Autodesk Inventor part; units mm, degrees
(part 2 of 6)
  arc A552 (-21.7306, 49.25) -> (-21.2315, 49.5618) centre (-21.7304, 49.805) ccw
  arc A553 (-21.2315, 49.5618) -> (-21.1389, 49.8696) centre (-22.1304, 50) ccw
  arc A554 (-20.9902, 50) -> (-21.1389, 49.8696) centre (-20.9902, 49.85) ccw
  line L94 (-20.9902, 50) -> (-20.4709, 50)
  arc A555 (-20.3222, 49.8696) -> (-20.4709, 50) centre (-20.4709, 49.85) ccw
  arc A556 (-20.3222, 49.8696) -> (-20.2296, 49.5618) centre (-19.3307, 50) ccw
  arc A557 (-20.2296, 49.5618) -> (-19.7306, 49.25) centre (-19.7307, 49.805) ccw
  arc A558 (-19.7306, 49.25) -> (-19.2315, 49.5618) centre (-19.7304, 49.805) ccw
  arc A559 (-19.2315, 49.5618) -> (-19.1389, 49.8696) centre (-20.1304, 50) ccw
  arc A560 (-18.9902, 50) -> (-19.1389, 49.8696) centre (-18.9902, 49.85) ccw
  line L95 (-18.9902, 50) -> (-18.4709, 50)
  arc A561 (-18.3222, 49.8696) -> (-18.4709, 50) centre (-18.4709, 49.85) ccw
  arc A562 (-18.3222, 49.8696) -> (-18.2296, 49.5618) centre (-17.3307, 50) ccw
  arc A563 (-18.2296, 49.5618) -> (-17.7306, 49.25) centre (-17.7307, 49.805) ccw
  arc A564 (-17.7306, 49.25) -> (-17.2315, 49.5618) centre (-17.7304, 49.805) ccw
  arc A565 (-17.2315, 49.5618) -> (-17.1389, 49.8696) centre (-18.1304, 50) ccw
  arc A566 (-16.9902, 50) -> (-17.1389, 49.8696) centre (-16.9902, 49.85) ccw
  line L96 (-16.9902, 50) -> (-16.4709, 50)
  arc A567 (-16.3222, 49.8696) -> (-16.4709, 50) centre (-16.4709, 49.85) ccw
  arc A568 (-16.3222, 49.8696) -> (-16.2296, 49.5618) centre (-15.3307, 50) ccw
  arc A569 (-16.2296, 49.5618) -> (-15.7306, 49.25) centre (-15.7307, 49.805) ccw
  arc A570 (-15.7306, 49.25) -> (-15.2315, 49.5618) centre (-15.7304, 49.805) ccw
  arc A571 (-15.2315, 49.5618) -> (-15.1389, 49.8696) centre (-16.1304, 50) ccw
  arc A572 (-14.9902, 50) -> (-15.1389, 49.8696) centre (-14.9902, 49.85) ccw
  line L97 (-14.9902, 50) -> (-14.4709, 50)
  arc A573 (-14.3222, 49.8696) -> (-14.4709, 50) centre (-14.4709, 49.85) ccw
  arc A574 (-14.3222, 49.8696) -> (-14.2296, 49.5618) centre (-13.3307, 50) ccw
  arc A575 (-14.2296, 49.5618) -> (-13.7306, 49.25) centre (-13.7307, 49.805) ccw
  arc A576 (-13.7306, 49.25) -> (-13.2315, 49.5618) centre (-13.7304, 49.805) ccw
  arc A577 (-13.2315, 49.5618) -> (-13.1389, 49.8696) centre (-14.1304, 50) ccw
  arc A578 (-12.9902, 50) -> (-13.1389, 49.8696) centre (-12.9902, 49.85) ccw
  line L98 (-12.9902, 50) -> (-12.4709, 50)
  arc A579 (-12.3222, 49.8696) -> (-12.4709, 50) centre (-12.4709, 49.85) ccw
  arc A580 (-12.3222, 49.8696) -> (-12.2296, 49.5618) centre (-11.3307, 50) ccw
  arc A581 (-12.2296, 49.5618) -> (-11.7306, 49.25) centre (-11.7307, 49.805) ccw
  arc A582 (-11.7306, 49.25) -> (-11.2315, 49.5618) centre (-11.7304, 49.805) ccw
  arc A583 (-11.2315, 49.5618) -> (-11.1389, 49.8696) centre (-12.1304, 50) ccw
  arc A584 (-10.9902, 50) -> (-11.1389, 49.8696) centre (-10.9902, 49.85) ccw
  line L99 (-10.9902, 50) -> (-10.4709, 50)
  arc A585 (-10.3222, 49.8696) -> (-10.4709, 50) centre (-10.4709, 49.85) ccw
  arc A586 (-10.3222, 49.8696) -> (-10.2296, 49.5618) centre (-9.3307, 50) ccw
  arc A587 (-10.2296, 49.5618) -> (-9.7306, 49.25) centre (-9.7307, 49.805) ccw
  arc A588 (-9.7306, 49.25) -> (-9.2315, 49.5618) centre (-9.7304, 49.805) ccw
  arc A589 (-9.2315, 49.5618) -> (-9.1389, 49.8696) centre (-10.1304, 50) ccw
  arc A590 (-8.9902, 50) -> (-9.1389, 49.8696) centre (-8.9902, 49.85) ccw
  line L100 (-8.9902, 50) -> (-8.4709, 50)
  arc A591 (-8.3222, 49.8696) -> (-8.4709, 50) centre (-8.4709, 49.85) ccw
  arc A592 (-8.3222, 49.8696) -> (-8.2296, 49.5618) centre (-7.3307, 50) ccw
  arc A593 (-8.2296, 49.5618) -> (-7.7306, 49.25) centre (-7.7307, 49.805) ccw
  arc A594 (-7.7306, 49.25) -> (-7.2315, 49.5618) centre (-7.7304, 49.805) ccw
  arc A595 (-7.2315, 49.5618) -> (-7.1389, 49.8696) centre (-8.1304, 50) ccw
  arc A596 (-6.9902, 50) -> (-7.1389, 49.8696) centre (-6.9902, 49.85) ccw
  line L101 (-6.9902, 50) -> (-6.4709, 50)
  arc A597 (-6.3222, 49.8696) -> (-6.4709, 50) centre (-6.4709, 49.85) ccw
  arc A598 (-6.3222, 49.8696) -> (-6.2296, 49.5618) centre (-5.3307, 50) ccw
  arc A599 (-6.2296, 49.5618) -> (-5.7306, 49.25) centre (-5.7307, 49.805) ccw
  arc A600 (-5.7306, 49.25) -> (-5.2315, 49.5618) centre (-5.7304, 49.805) ccw
  arc A601 (-5.2315, 49.5618) -> (-5.1389, 49.8696) centre (-6.1304, 50) ccw
  arc A602 (-4.9902, 50) -> (-5.1389, 49.8696) centre (-4.9902, 49.85) ccw
  line L102 (-4.9902, 50) -> (-4.4709, 50)
  arc A603 (-4.3222, 49.8696) -> (-4.4709, 50) centre (-4.4709, 49.85) ccw
  arc A604 (-4.3222, 49.8696) -> (-4.2296, 49.5618) centre (-3.3307, 50) ccw
  arc A605 (-4.2296, 49.5618) -> (-3.7306, 49.25) centre (-3.7307, 49.805) ccw
  arc A606 (-3.7306, 49.25) -> (-3.2315, 49.5618) centre (-3.7304, 49.805) ccw
  arc A607 (-3.2315, 49.5618) -> (-3.1389, 49.8696) centre (-4.1304, 50) ccw
  arc A608 (-2.9902, 50) -> (-3.1389, 49.8696) centre (-2.9902, 49.85) ccw
  line L103 (-2.9902, 50) -> (-2.4709, 50)
  arc A609 (-2.3222, 49.8696) -> (-2.4709, 50) centre (-2.4709, 49.85) ccw
  arc A610 (-2.3222, 49.8696) -> (-2.2296, 49.5618) centre (-1.3307, 50) ccw
  arc A611 (-2.2296, 49.5618) -> (-1.7306, 49.25) centre (-1.7307, 49.805) ccw
  arc A612 (-1.7306, 49.25) -> (-1.2315, 49.5618) centre (-1.7304, 49.805) ccw
  arc A613 (-1.2315, 49.5618) -> (-1.1389, 49.8696) centre (-2.1304, 50) ccw
  arc A614 (-0.9902, 50) -> (-1.1389, 49.8696) centre (-0.9902, 49.85) ccw
  line L104 (-0.9902, 50) -> (-0.3754, 50)
  arc A615 (-0.3433, 49.9187) -> (-0.3754, 50) centre (-0.4928, 49.9067) ccw
  arc A616 (-0.3433, 49.9187) -> (-0.2664, 49.6066) centre (0.6535, 49.9986) ccw
  arc A617 (-0.2664, 49.6066) -> (0.2388, 49.2692) centre (0.2441, 49.8242) ccw
  arc A618 (0.2388, 49.2692) -> (0.7304, 49.556) centre (0.2445, 49.8242) ccw
  arc A619 (0.7304, 49.556) -> (0.8385, 49.8586) centre (-0.1451, 50.0392) ccw
  arc A620 (0.9717, 49.9809) -> (0.8385, 49.8586) centre (0.986, 49.8316) ccw
  arc A621 (1.534, 49.9523) -> (0.9717, 49.9809) centre (0, 25.315) ccw
  arc A622 (1.6541, 49.8172) -> (1.534, 49.9523) centre (1.5046, 49.8052) ccw
  arc A623 (1.6541, 49.8172) -> (1.731, 49.5051) centre (2.6509, 49.8971) ccw
  arc A624 (1.731, 49.5051) -> (2.191, 49.17) centre (2.2415, 49.7227) ccw
  arc A625 (2.191, 49.17) -> (2.7278, 49.4544) centre (2.2419, 49.7227) ccw
  arc A626 (2.7278, 49.4544) -> (2.8359, 49.7571) centre (1.8523, 49.9377) ccw
  arc A627 (2.8736, 49.8322) -> (2.8359, 49.7571) centre (2.9834, 49.73) ccw
  arc A628 (3.5639, 49.7414) -> (2.8736, 49.8322) centre (0, 25.315) ccw
  arc A629 (3.5809, 49.6591) -> (3.5639, 49.7414) centre (3.4314, 49.6711) ccw
  arc A630 (3.5809, 49.6591) -> (3.6071, 49.3388) centre (4.5777, 49.5792) ccw
  arc A631 (3.6071, 49.3388) -> (4.0521, 48.9252) centre (4.1458, 49.4722) ccw
  arc A632 (4.0521, 48.9252) -> (4.5831, 49.13) centre (4.1461, 49.4722) ccw
  arc A633 (4.5831, 49.13) -> (4.738, 49.4116) centre (3.7958, 49.7466) ccw
  arc A634 (4.889, 49.511) -> (4.738, 49.4116) centre (4.8793, 49.3613) ccw
  arc A635 (5.4396, 49.3932) -> (4.889, 49.511) centre (0, 25.315) ccw
  arc A636 (5.5366, 49.2407) -> (5.4396, 49.3932) centre (5.3871, 49.2527) ccw
  arc A637 (5.5366, 49.2407) -> (5.5628, 48.9204) centre (6.5335, 49.1608) ccw
  arc A638 (5.5628, 48.9204) -> (5.9635, 48.5162) centre (6.1015, 49.0538) ccw
  arc A639 (5.9635, 48.5162) -> (6.5388, 48.7115) centre (6.1019, 49.0537) ccw
  arc A640 (6.5388, 48.7115) -> (6.6937, 48.9931) centre (5.7515, 49.3281) ccw
  arc A641 (6.7429, 49.0612) -> (6.6937, 48.9931) centre (6.8351, 48.9429) ccw
  arc A642 (7.41, 48.8616) -> (6.7429, 49.0612) centre (0, 25.315) ccw
  arc A643 (7.4136, 48.7777) -> (7.41, 48.8616) centre (7.2679, 48.8133) ccw
  arc A644 (7.4136, 48.7777) -> (7.3884, 48.4573) centre (8.385, 48.54) ccw
  arc A645 (7.3884, 48.4573) -> (7.7618, 47.9781) centre (7.9415, 48.5032) ccw
  arc A646 (7.7618, 47.9781) -> (8.3187, 48.0956) centre (7.9418, 48.5031) ccw
  arc A647 (8.3187, 48.0956) -> (8.5165, 48.3489) centre (7.6397, 48.8298) ccw
  arc A648 (8.6814, 48.4231) -> (8.5165, 48.3489) centre (8.648, 48.2768) ccw
  arc A649 (9.2062, 48.219) -> (8.6814, 48.4231) centre (0, 25.315) ccw
  arc A650 (9.2777, 48.053) -> (9.2062, 48.219) centre (9.132, 48.0887) ccw
  arc A651 (9.2777, 48.053) -> (9.2525, 47.7326) centre (10.2491, 47.8153) ccw
  arc A652 (9.2525, 47.7326) -> (9.5837, 47.2698) centre (9.8056, 47.7785) ccw
  arc A653 (9.5837, 47.2698) -> (10.1828, 47.3709) centre (9.8059, 47.7784) ccw
  arc A654 (10.1828, 47.3709) -> (10.3806, 47.6243) centre (9.5038, 48.1051) ccw
  arc A655 (10.44, 47.6836) -> (10.3806, 47.6243) centre (10.5121, 47.5521) ccw
  arc A656 (11.0667, 47.3803) -> (10.44, 47.6836) centre (0, 25.315) ccw
  arc A657 (11.057, 47.2969) -> (11.0667, 47.3803) centre (10.9188, 47.3553) ccw
  arc A658 (11.057, 47.2969) -> (10.981, 46.9846) centre (11.978, 46.9075) ccw
  arc A659 (10.981, 46.9846) -> (11.2734, 46.452) centre (11.5344, 46.9418) ccw
  arc A660 (11.2734, 46.452) -> (11.8418, 46.4794) centre (11.5347, 46.9416) ccw
  arc A661 (11.8418, 46.4794) -> (12.0775, 46.6979) centre (11.2884, 47.3123) ccw
  arc A662 (12.252, 46.7448) -> (12.0775, 46.6979) centre (12.1958, 46.6058) ccw
  arc A663 (12.7377, 46.4598) -> (12.252, 46.7448) centre (0, 25.315) ccw
  arc A664 (12.7818, 46.2845) -> (12.7377, 46.4598) centre (12.6436, 46.3429) ccw
  arc A665 (12.7818, 46.2845) -> (12.7059, 45.9722) centre (13.7029, 45.8951) ccw
  arc A666 (12.7059, 45.9722) -> (12.9591, 45.4625) centre (13.2592, 45.9294) ccw
  arc A667 (12.9591, 45.4625) -> (13.5666, 45.4669) centre (13.2595, 45.9292) ccw
  arc A668 (13.5666, 45.4669) -> (13.8023, 45.6855) centre (13.0133, 46.2999) ccw
  arc A669 (13.8704, 45.7347) -> (13.8023, 45.6855) centre (13.9206, 45.5933) ccw
  arc A670 (14.4408, 45.3353) -> (13.8704, 45.7347) centre (0, 25.315) ccw
  arc A671 (14.4179, 45.2545) -> (14.4408, 45.3353) centre (14.2908, 45.3342) ccw
  arc A672 (14.4179, 45.2545) -> (14.2931, 44.9583) centre (15.2651, 44.7234) ccw
  arc A673 (14.2931, 44.9583) -> (14.4969, 44.386) centre (14.8326, 44.8279) ccw
  arc A674 (14.4969, 44.386) -> (15.0624, 44.3224) centre (14.8329, 44.8277) ccw
  arc A675 (15.0624, 44.3224) -> (15.3299, 44.5006) centre (14.6488, 45.2329) ccw
  arc A676 (15.5097, 44.5191) -> (15.3299, 44.5006) centre (15.432, 44.3908) ccw
  arc A677 (15.9437, 44.1604) -> (15.5097, 44.5191) centre (0, 25.315) ccw
  arc A678 (15.9594, 43.9803) -> (15.9437, 44.1604) centre (15.8323, 44.0599) ccw
  arc A679 (15.9594, 43.9803) -> (15.8346, 43.6841) centre (16.8066, 43.4491) ccw
  arc A680 (15.8346, 43.6841) -> (16.0035, 43.1406) centre (16.3741, 43.5537) ccw
  arc A681 (16.0035, 43.1406) -> (16.6039, 43.0481) centre (16.3744, 43.5534) ccw
  arc A682 (16.6039, 43.0481) -> (16.8714, 43.2263) centre (16.1903, 43.9586) ccw
  arc A683 (16.9464, 43.264) -> (16.8714, 43.2263) centre (16.9735, 43.1165) ccw
  arc A684 (17.4459, 42.7789) -> (16.9464, 43.264) centre (0, 25.315) ccw
  arc A685 (17.4104, 42.7028) -> (17.4459, 42.7789) centre (17.2977, 42.8017) ccw
  arc A686 (17.4104, 42.7028) -> (17.2401, 42.4303) centre (18.1623, 42.0435) ccw
  arc A687 (17.2401, 42.4303) -> (17.3501, 41.8328) centre (17.7519, 42.2156) ccw
  arc A688 (17.3501, 41.8328) -> (17.8983, 41.6799) centre (17.7522, 42.2153) ccw
  arc A689 (17.8983, 41.6799) -> (18.1907, 41.8132) centre (17.635, 42.6446) ccw
  arc A690 (18.3712, 41.8029) -> (18.1907, 41.8132) centre (18.274, 41.6885) ccw
  arc A691 (18.7425, 41.3795) -> (18.3712, 41.8029) centre (0, 25.315) ccw
  arc A692 (18.7292, 41.1992) -> (18.7425, 41.3795) centre (18.6165, 41.2981) ccw
  arc A693 (18.7292, 41.1992) -> (18.5589, 40.9267) centre (19.4811, 40.5399) ccw
  arc A694 (18.5589, 40.9267) -> (18.639, 40.3632) centre (19.0707, 40.712) ccw
  arc A695 (18.639, 40.3632) -> (19.2171, 40.1763) centre (19.0709, 40.7117) ccw
  arc A696 (19.2171, 40.1763) -> (19.5095, 40.3097) centre (18.9538, 41.141) ccw
  arc A697 (19.5896, 40.3349) -> (19.5095, 40.3097) centre (19.5928, 40.1849) ccw
  arc A698 (20.0054, 39.7764) -> (19.5896, 40.3349) centre (0, 25.315) ccw
  arc A699 (19.9583, 39.7069) -> (20.0054, 39.7764) centre (19.8627, 39.8225) ccw
  arc A700 (19.9583, 39.7069) -> (19.7467, 39.465) centre (20.5954, 38.9362) ccw
  arc A701 (19.7467, 39.465) -> (19.76, 38.8576) centre (20.2177, 39.1715) ccw
  arc A702 (19.76, 38.8576) -> (20.2769, 38.6194) centre (20.2179, 39.1712) ccw
  arc A703 (20.2769, 38.6194) -> (20.5868, 38.7044) centre (20.1707, 39.6137) ccw
  arc A704 (20.7633, 38.6654) -> (20.5868, 38.7044) centre (20.6492, 38.568) ccw
  arc A705 (21.0624, 38.1883) -> (20.7633, 38.6654) centre (0, 25.315) ccw
  arc A706 (21.0207, 38.0124) -> (21.0624, 38.1883) centre (20.9251, 38.1281) ccw
  arc A707 (21.0207, 38.0124) -> (20.8091, 37.7705) centre (21.6578, 37.2417) ccw
  arc A708 (20.8091, 37.7705) -> (20.7984, 37.2015) centre (21.2802, 37.477) ccw
  arc A709 (20.7984, 37.2015) -> (21.3393, 36.9249) centre (21.2803, 37.4767) ccw
  arc A710 (21.3393, 36.9249) -> (21.6492, 37.0099) centre (21.2331, 37.9192) ccw
  arc A711 (21.7323, 37.0221) -> (21.6492, 37.0099) centre (21.7116, 36.8735) ccw
  arc A712 (22.0539, 36.4045) -> (21.7323, 37.0221) centre (0, 25.315) ccw
  arc A713 (21.9962, 36.3434) -> (22.0539, 36.4045) centre (21.9203, 36.4728) ccw
  arc A714 (21.9962, 36.3434) -> (21.7488, 36.1383) centre (22.5025, 35.481) ccw
  arc A715 (21.7488, 36.1383) -> (21.6652, 35.5365) centre (22.1671, 35.7735) ccw
  arc A716 (21.6652, 35.5365) -> (22.1375, 35.219) centre (22.1673, 35.7732) ccw
  arc A717 (22.1375, 35.219) -> (22.457, 35.2535) centre (22.1911, 36.2175) ccw
  arc A718 (22.6251, 35.1869) -> (22.457, 35.2535) centre (22.4969, 35.1089) ccw
  arc A719 (22.8444, 34.6683) -> (22.6251, 35.1869) centre (0, 25.315) ccw
  arc A720 (22.7751, 34.5013) -> (22.8444, 34.6683) centre (22.6992, 34.6306) ccw
  arc A721 (22.7751, 34.5013) -> (22.5277, 34.2962) centre (23.2814, 33.6389) ccw
  arc A722 (22.5277, 34.2962) -> (22.4265, 33.7361) centre (22.946, 33.9314) ccw
  arc A723 (22.4265, 33.7361) -> (22.9164, 33.3768) centre (22.9461, 33.931) ccw
  arc A724 (22.9164, 33.3768) -> (23.2359, 33.4114) centre (22.9699, 34.3754) ccw
  arc A725 (23.3199, 33.4102) -> (23.2359, 33.4114) centre (23.2758, 33.2668) ccw
  arc A726 (23.5389, 32.7493) -> (23.3199, 33.4102) centre (0, 25.315) ccw
  arc A727 (23.4723, 32.6981) -> (23.5389, 32.7493) centre (23.4179, 32.8379) ccw
  arc A728 (23.4723, 32.6981) -> (23.1954, 32.535) centre (23.8347, 31.7661) ccw
  arc A729 (23.1954, 32.535) -> (23.017, 31.9543) centre (23.5502, 32.1083) ccw
  arc A730 (23.017, 31.9543) -> (23.4326, 31.5655) centre (23.5503, 32.1079) ccw
  arc A731 (23.4326, 31.5655) -> (23.7536, 31.5488) centre (23.6446, 32.5428) ccw
  arc A732 (23.9089, 31.4562) -> (23.7536, 31.5488) centre (23.7699, 31.3997) ccw
  arc A733 (24.0427, 30.9093) -> (23.9089, 31.4562) centre (0, 25.315) ccw
  arc A734 (23.9478, 30.7555) -> (24.0427, 30.9093) centre (23.8934, 30.8953) ccw
  arc A735 (23.9478, 30.7555) -> (23.6708, 30.5924) centre (24.3101, 29.8234) ccw
  arc A736 (23.6708, 30.5924) -> (23.4817, 30.0556) centre (24.0256, 30.1656) ccw
  arc A737 (23.4817, 30.0556) -> (23.9081, 29.6229) centre (24.0257, 30.1653) ccw
  arc A738 (23.9081, 29.6229) -> (24.229, 29.6061) centre (24.12, 30.6002) ccw
  arc A739 (24.3117, 29.5915) -> (24.229, 29.6061) centre (24.2454, 29.457) ccw
  arc A740 (24.4227, 28.9041) -> (24.3117, 29.5915) centre (0, 25.315) ccw
  arc A741 (24.3488, 28.8643) -> (24.4227, 28.9041) centre (24.3174, 29.0109) ccw
  arc A742 (24.3488, 28.8643) -> (24.0494, 28.7474) centre (24.558, 27.8864) ccw
  arc A743 (24.0494, 28.7474) -> (23.7808, 28.2025) centre (24.3317, 28.2695) ccw
  arc A744 (23.7808, 28.2025) -> (24.1292, 27.7525) centre (24.3317, 28.2692) ccw
  arc A745 (24.1292, 27.7525) -> (24.4434, 27.6848) centre (24.4941, 28.6835) ccw
  arc A746 (24.5819, 27.5687) -> (24.4434, 27.6848) centre (24.4357, 27.535) ccw
  arc A747 (24.6269, 27.0074) -> (24.5819, 27.5687) centre (0, 25.315) ccw
  arc A748 (24.5086, 26.8707) -> (24.6269, 27.0074) centre (24.4772, 27.0173) ccw
  arc A749 (24.5086, 26.8707) -> (24.2093, 26.7538) centre (24.7179, 25.8928) ccw
  arc A750 (24.2093, 26.7538) -> (23.937, 26.254) centre (24.4916, 26.2759) ccw
  arc A751 (23.937, 26.254) -> (24.289, 25.7589) centre (24.4916, 26.2756) ccw
  arc A752 (24.289, 25.7589) -> (24.6032, 25.6912) centre (24.654, 26.6899) ccw
  arc A753 (24.6825, 25.6636) -> (24.6032, 25.6912) centre (24.5956, 25.5414) ccw
  arc A754 (24.6826, 24.9673) -> (24.6825, 25.6636) centre (0, 25.315) ccw
  arc A755 (24.6032, 24.9397) -> (24.6826, 24.9673) centre (24.5956, 25.0895) ccw
  arc A756 (24.6032, 24.9397) -> (24.289, 24.872) centre (24.654, 23.941) ccw
  arc A757 (24.289, 24.872) -> (23.937, 24.3769) centre (24.4916, 24.3553) ccw
  arc A758 (23.937, 24.3769) -> (24.2093, 23.8771) centre (24.4916, 24.355) ccw
  arc A759 (24.2093, 23.8771) -> (24.5087, 23.7602) centre (24.7179, 24.7381) ccw
  arc A760 (24.627, 23.6235) -> (24.5087, 23.7602) centre (24.4773, 23.6136) ccw
  arc A761 (24.582, 23.0622) -> (24.627, 23.6235) centre (0, 25.315) ccw
  arc A762 (24.4434, 22.9461) -> (24.582, 23.0622) centre (24.4358, 23.0959) ccw
  arc A763 (24.4434, 22.9461) -> (24.1293, 22.8784) centre (24.4943, 21.9474) ccw
  arc A764 (24.1293, 22.8784) -> (23.7809, 22.4284) centre (24.3318, 22.3617) ccw
  arc A765 (23.7809, 22.4284) -> (24.0495, 21.8835) centre (24.3318, 22.3614) ccw
  arc A766 (24.0495, 21.8835) -> (24.3489, 21.7666) centre (24.5581, 22.7445) ccw
  arc A767 (24.4228, 21.7268) -> (24.3489, 21.7666) centre (24.3175, 21.62) ccw
  arc A768 (24.3119, 21.0394) -> (24.4228, 21.7268) centre (0, 25.315) ccw
  arc A769 (24.2292, 21.0248) -> (24.3119, 21.0394) centre (24.2455, 21.1739) ccw
  arc A770 (24.2292, 21.0248) -> (23.9082, 21.008) centre (24.1202, 20.0307) ccw
  arc A771 (23.9082, 21.008) -> (23.4818, 20.5753) centre (24.0259, 20.4656) ccw
  arc A772 (23.4818, 20.5753) -> (23.671, 20.0385) centre (24.0258, 20.4653) ccw
  arc A773 (23.671, 20.0385) -> (23.948, 19.8754) centre (24.3103, 20.8075) ccw
  arc A774 (24.0429, 19.7216) -> (23.948, 19.8754) centre (23.8936, 19.7356) ccw
  arc A775 (23.9091, 19.1747) -> (24.0429, 19.7216) centre (0, 25.315) ccw
  arc A776 (23.7538, 19.0821) -> (23.9091, 19.1747) centre (23.7702, 19.2312) ccw
  arc A777 (23.7538, 19.0821) -> (23.4329, 19.0653) centre (23.6449, 18.088) ccw
  arc A778 (23.4329, 19.0653) -> (23.0172, 18.6766) centre (23.5505, 18.5229) ccw
  arc A779 (23.0172, 18.6766) -> (23.1956, 18.0958) centre (23.5504, 18.5226) ccw
  arc A780 (23.1956, 18.0958) -> (23.4726, 17.9327) centre (23.8349, 18.8648) ccw
  arc A781 (23.5392, 17.8816) -> (23.4726, 17.9327) centre (23.4182, 17.7929) ccw
  arc A782 (23.3202, 17.2207) -> (23.5392, 17.8816) centre (0, 25.315) ccw
  arc A783 (23.2362, 17.2194) -> (23.3202, 17.2207) centre (23.2761, 17.364) ccw
  arc A784 (23.2362, 17.2194) -> (22.9167, 17.254) centre (22.9703, 16.2554) ccw
  arc A785 (22.9167, 17.254) -> (22.4268, 16.8947) centre (22.9464, 16.6998) ccw
  arc A786 (22.4268, 16.8947) -> (22.528, 16.3347) centre (22.9463, 16.6995) ccw
  arc A787 (22.528, 16.3347) -> (22.7754, 16.1295) centre (23.2817, 16.992) ccw
  arc A788 (22.8447, 15.9626) -> (22.7754, 16.1295) centre (22.6995, 16.0002) ccw
  arc A789 (22.6255, 15.4439) -> (22.8447, 15.9626) centre (0, 25.315) ccw
  arc A790 (22.4574, 15.3773) -> (22.6255, 15.4439) centre (22.4973, 15.5219) ccw
  arc A791 (22.4574, 15.3773) -> (22.1379, 15.4119) centre (22.1915, 14.4133) ccw
  arc A792 (22.1379, 15.4119) -> (21.6656, 15.0943) centre (22.1676, 14.8577) ccw
  arc A793 (21.6656, 15.0943) -> (21.7492, 14.4925) centre (22.1675, 14.8573) ccw
  arc A794 (21.7492, 14.4925) -> (21.9966, 14.2874) centre (22.5029, 15.1498) ccw
  arc A795 (22.0543, 14.2263) -> (21.9966, 14.2874) centre (21.9207, 14.1581) ccw
  arc A796 (21.7327, 13.6087) -> (22.0543, 14.2263) centre (0, 25.315) ccw
  arc A797 (21.6496, 13.6209) -> (21.7327, 13.6087) centre (21.7121, 13.7573) ccw
  arc A798 (21.6496, 13.6209) -> (21.3397, 13.7059) centre (21.2335, 12.7116) ccw
  arc A799 (21.3397, 13.7059) -> (20.7988, 13.4293) centre (21.2808, 13.1541) ccw
  arc A800 (20.7988, 13.4293) -> (20.8096, 12.8602) centre (21.2806, 13.1537) ccw
  arc A801 (20.8096, 12.8602) -> (21.0211, 12.6183) centre (21.6583, 13.3891) ccw
  arc A802 (21.0629, 12.4424) -> (21.0211, 12.6183) centre (20.9256, 12.5027) ccw
  arc A803 (20.7638, 11.9654) -> (21.0629, 12.4424) centre (0, 25.315) ccw
  arc A804 (20.5873, 11.9263) -> (20.7638, 11.9654) centre (20.6497, 12.0627) ccw
  arc A805 (20.5873, 11.9263) -> (20.2774, 12.0114) centre (20.1712, 11.017) ccw
  arc A806 (20.2774, 12.0114) -> (19.7605, 11.7731) centre (20.2184, 11.4595) ccw
  arc A807 (19.7605, 11.7731) -> (19.7472, 11.1657) centre (20.2182, 11.4592) ccw
  arc A808 (19.7472, 11.1657) -> (19.9588, 10.9238) centre (20.5959, 11.6945) ccw
  arc A809 (20.0059, 10.8543) -> (19.9588, 10.9238) centre (19.8632, 10.8082) ccw
  arc A810 (19.5901, 10.2958) -> (20.0059, 10.8543) centre (0, 25.315) ccw
  arc A811 (19.51, 10.3211) -> (19.5901, 10.2958) centre (19.5934, 10.4458) ccw
  arc A812 (19.51, 10.3211) -> (19.2176, 10.4544) centre (18.9544, 9.4897) ccw
  arc A813 (19.2176, 10.4544) -> (18.6395, 10.2674) centre (19.0715, 9.919) ccw
  arc A814 (18.6395, 10.2674) -> (18.5595, 9.704) centre (19.0713, 9.9187) ccw
  arc A815 (18.5595, 9.704) -> (18.7298, 9.4314) centre (19.4816, 10.0908) ccw
  arc A816 (18.7431, 9.2512) -> (18.7298, 9.4314) centre (18.6171, 9.3325) ccw
  arc A817 (18.3718, 8.8278) -> (18.7431, 9.2512) centre (0, 25.315) ccw
  arc A818 (18.1913, 8.8174) -> (18.3718, 8.8278) centre (18.2747, 8.9421) ccw
  arc A819 (18.1913, 8.8174) -> (17.8989, 8.9507) centre (17.6356, 7.986) ccw
  arc A820 (17.8989, 8.9507) -> (17.3507, 8.7979) centre (17.7528, 8.4153) ccw
  arc A821 (17.3507, 8.7979) -> (17.2407, 8.2004) centre (17.7525, 8.4151) ccw
  arc A822 (17.2407, 8.2004) -> (17.4111, 7.9278) centre (18.1629, 8.5872) ccw
  arc A823 (17.4466, 7.8517) -> (17.4111, 7.9278) centre (17.2983, 7.8289) ccw
  arc A824 (16.9471, 7.3666) -> (17.4466, 7.8517) centre (0, 25.315) ccw
  arc A825 (16.872, 7.4043) -> (16.9471, 7.3666) centre (16.9742, 7.5141) ccw
  arc A826 (16.872, 7.4043) -> (16.6046, 7.5825) centre (16.191, 6.672) ccw
  arc A827 (16.6046, 7.5825) -> (16.0041, 7.49) centre (16.375, 7.0772) ccw
  arc A828 (16.0041, 7.49) -> (15.8353, 6.9465) centre (16.3748, 7.0769) ccw
  arc A829 (15.8353, 6.9465) -> (15.9601, 6.6503) centre (16.8073, 7.1815) ccw
  arc A830 (15.9444, 6.4702) -> (15.9601, 6.6503) centre (15.833, 6.5706) ccw
  arc A831 (15.5104, 6.1114) -> (15.9444, 6.4702) centre (0, 25.315) ccw
  arc A832 (15.3306, 6.1299) -> (15.5104, 6.1114) centre (15.4327, 6.2398) ccw
  arc A833 (15.3306, 6.1299) -> (15.0631, 6.3081) centre (14.6496, 5.3977) ccw
  arc A834 (15.0631, 6.3081) -> (14.4976, 6.2446) centre (14.8336, 5.8028) ccw
  arc A835 (14.4976, 6.2446) -> (14.2938, 5.6722) centre (14.8333, 5.8026) ccw
  arc A836 (14.2938, 5.6722) -> (14.4186, 5.376) centre (15.2658, 5.9072) ccw
  arc A837 (14.4415, 5.2952) -> (14.4186, 5.376) centre (14.2915, 5.2963) ccw
  arc A838 (13.8711, 4.8959) -> (14.4415, 5.2952) centre (0, 25.315) ccw
  arc A839 (13.803, 4.945) -> (13.8711, 4.8959) centre (13.9214, 5.0372) ccw
  arc A840 (13.803, 4.945) -> (13.5674, 5.1636) centre (13.014, 4.3306) ccw
  arc A841 (13.5674, 5.1636) -> (12.9599, 5.168) centre (13.2603, 4.7013) ccw
  arc A842 (12.9599, 5.168) -> (12.7066, 4.6583) centre (13.26, 4.7011) ccw
  arc A843 (12.7066, 4.6583) -> (12.7826, 4.346) centre (13.7036, 4.7354) ccw
  arc A844 (12.7384, 4.1707) -> (12.7826, 4.346) centre (12.6444, 4.2876) ccw
  arc A845 (12.2528, 3.8856) -> (12.7384, 4.1707) centre (0, 25.315) ccw
  arc A846 (12.0782, 3.9325) -> (12.2528, 3.8856) centre (12.1966, 4.0247) ccw
  arc A847 (12.0782, 3.9325) -> (11.8426, 4.1511) centre (11.2892, 3.3181) ccw
  arc A848 (11.8426, 4.1511) -> (11.2741, 4.1784) centre (11.5355, 3.6888) ccw
  arc A849 (11.2741, 4.1784) -> (10.9818, 3.6458) centre (11.5352, 3.6886) ccw
  arc A850 (10.9818, 3.6458) -> (11.0578, 3.3335) centre (11.9788, 3.723) ccw
  arc A851 (11.0675, 3.2501) -> (11.0578, 3.3335) centre (10.9196, 3.2751) ccw
  arc A852 (10.4408, 2.9467) -> (11.0675, 3.2501) centre (0, 25.315) ccw
  arc A853 (10.3814, 3.0061) -> (10.4408, 2.9467) centre (10.5129, 3.0783) ccw
  arc A854 (10.3814, 3.0061) -> (10.1836, 3.2594) centre (9.5046, 2.5253) ccw
  arc A855 (10.1836, 3.2594) -> (9.5845, 3.3605) centre (9.8068, 2.852) ccw
  arc A856 (9.5845, 3.3605) -> (9.2533, 2.8977) centre (9.8064, 2.8518) ccw
  arc A857 (9.2533, 2.8977) -> (9.2786, 2.5773) centre (10.2499, 2.815) ccw
  arc A858 (9.2071, 2.4113) -> (9.2786, 2.5773) centre (9.1329, 2.5417) ccw
  arc A859 (8.6822, 2.2073) -> (9.2071, 2.4113) centre (0, 25.315) ccw
  arc A860 (8.5174, 2.2814) -> (8.6822, 2.2073) centre (8.6489, 2.3535) ccw
  arc A861 (8.5174, 2.2814) -> (8.3195, 2.5347) centre (7.6406, 1.8005) ccw
  arc A862 (8.3195, 2.5347) -> (7.7627, 2.6522) centre (7.9427, 2.1272) ccw
  arc A863 (7.7627, 2.6522) -> (7.3893, 2.173) centre (7.9424, 2.1271) ccw
  arc A864 (7.3893, 2.173) -> (7.4145, 1.8526) centre (8.3858, 2.0903) ccw
  arc A865 (7.4108, 1.7687) -> (7.4145, 1.8526) centre (7.2688, 1.8169) ccw
  arc A866 (6.7438, 1.569) -> (7.4108, 1.7687) centre (0, 25.315) ccw
  arc A867 (6.6946, 1.6371) -> (6.7438, 1.569) centre (6.8359, 1.6874) ccw
  arc A868 (6.6946, 1.6371) -> (6.5397, 1.9187) centre (5.7524, 1.3021) ccw
  arc A869 (6.5397, 1.9187) -> (5.9644, 2.114) centre (6.1027, 1.5765) ccw
  arc A870 (5.9644, 2.114) -> (5.5637, 1.7098) centre (6.1024, 1.5764) ccw
  arc A871 (5.5637, 1.7098) -> (5.5375, 1.3895) centre (6.5343, 1.4694) ccw
  arc A872 (5.4405, 1.237) -> (5.5375, 1.3895) centre (5.388, 1.3775) ccw
  arc A873 (4.8899, 1.1192) -> (5.4405, 1.237) centre (0, 25.315) ccw
  arc A874 (4.7389, 1.2186) -> (4.8899, 1.1192) centre (4.8802, 1.2689) ccw
  arc A875 (4.7389, 1.2186) -> (4.5839, 1.5002) centre (3.7967, 0.8836) ccw
  arc A876 (4.5839, 1.5002) -> (4.0529, 1.7049) centre (4.147, 1.158) ccw
  arc A877 (4.0529, 1.7049) -> (3.6079, 1.2913) centre (4.1467, 1.1579) ccw
  arc A878 (3.6079, 1.2913) -> (3.5818, 0.971) centre (4.5786, 1.0509) ccw
  arc A879 (3.5648, 0.8888) -> (3.5818, 0.971) centre (3.4323, 0.959) ccw
  arc A880 (2.8745, 0.7979) -> (3.5648, 0.8888) centre (0, 25.315) ccw
  arc A881 (2.8368, 0.873) -> (2.8745, 0.7979) centre (2.9843, 0.9001) ccw
  arc A882 (2.8368, 0.873) -> (2.7287, 1.1757) centre (1.8532, 0.6924) ccw
  arc A883 (2.7287, 1.1757) -> (2.1918, 1.4601) centre (2.2428, 0.9074) ccw
  arc A884 (2.1918, 1.4601) -> (1.7319, 1.1249) centre (2.2424, 0.9074) ccw
  arc A885 (1.7319, 1.1249) -> (1.655, 0.8129) centre (2.6518, 0.733) ccw
  arc A886 (1.5349, 0.6778) -> (1.655, 0.8129) centre (1.5055, 0.8249) ccw
  arc A887 (0.9726, 0.6492) -> (1.5349, 0.6778) centre (0, 25.315) ccw
  arc A888 (0.8394, 0.7714) -> (0.9726, 0.6492) centre (0.9869, 0.7985) ccw
  arc A889 (0.8394, 0.7714) -> (0.7313, 1.0741) centre (-0.1442, 0.5908) ccw
  arc A890 (0.7313, 1.0741) -> (0.2397, 1.3608) centre (0.2454, 0.8058) ccw
  arc A891 (0.2397, 1.3608) -> (-0.2656, 1.0234) centre (0.245, 0.8058) ccw
  arc A892 (-0.2656, 1.0234) -> (-0.3424, 0.7113) centre (0.6544, 0.6314) ccw
  arc A893 (-0.3744, 0.63) -> (-0.3424, 0.7113) centre (-0.4919, 0.7233) ccw
  line L105 (-0.3744, 0.63) -> (-0.9893, 0.63)
  arc A894 (-1.138, 0.7604) -> (-0.9893, 0.63) centre (-0.9893, 0.78) ccw
  arc A895 (-1.138, 0.7604) -> (-1.2306, 1.0682) centre (-2.1294, 0.63) ccw
  arc A896 (-1.2306, 1.0682) -> (-1.7296, 1.38) centre (-1.7294, 0.825) ccw
  arc A897 (-1.7296, 1.38) -> (-2.2287, 1.0682) centre (-1.7298, 0.825) ccw
  arc A898 (-2.2287, 1.0682) -> (-2.3213, 0.7604) centre (-1.3298, 0.63) ccw
  arc A899 (-2.47, 0.63) -> (-2.3213, 0.7604) centre (-2.47, 0.78) ccw
  line L106 (-2.47, 0.63) -> (-2.9893, 0.63)
  arc A900 (-3.138, 0.7604) -> (-2.9893, 0.63) centre (-2.9893, 0.78) ccw
  arc A901 (-3.138, 0.7604) -> (-3.2306, 1.0682) centre (-4.1294, 0.63) ccw
  arc A902 (-3.2306, 1.0682) -> (-3.7296, 1.38) centre (-3.7294, 0.825) ccw
  arc A903 (-3.7296, 1.38) -> (-4.2287, 1.0682) centre (-3.7298, 0.825) ccw
  arc A904 (-4.2287, 1.0682) -> (-4.3213, 0.7604) centre (-3.3298, 0.63) ccw
  arc A905 (-4.47, 0.63) -> (-4.3213, 0.7604) centre (-4.47, 0.78) ccw
  line L107 (-4.47, 0.63) -> (-4.9893, 0.63)
  arc A906 (-5.138, 0.7604) -> (-4.9893, 0.63) centre (-4.9893, 0.78) ccw
  arc A907 (-5.138, 0.7604) -> (-5.2306, 1.0682) centre (-6.1294, 0.63) ccw
  arc A908 (-5.2306, 1.0682) -> (-5.7296, 1.38) centre (-5.7294, 0.825) ccw
  arc A909 (-5.7296, 1.38) -> (-6.2287, 1.0682) centre (-5.7298, 0.825) ccw
  arc A910 (-6.2287, 1.0682) -> (-6.3213, 0.7604) centre (-5.3298, 0.63) ccw
  arc A911 (-6.47, 0.63) -> (-6.3213, 0.7604) centre (-6.47, 0.78) ccw
  line L108 (-6.47, 0.63) -> (-6.9893, 0.63)
  arc A912 (-7.138, 0.7604) -> (-6.9893, 0.63) centre (-6.9893, 0.78) ccw
  arc A913 (-7.138, 0.7604) -> (-7.2306, 1.0682) centre (-8.1294, 0.63) ccw
  arc A914 (-7.2306, 1.0682) -> (-7.7296, 1.38) centre (-7.7294, 0.825) ccw
  arc A915 (-7.7296, 1.38) -> (-8.2287, 1.0682) centre (-7.7298, 0.825) ccw
  arc A916 (-8.2287, 1.0682) -> (-8.3213, 0.7604) centre (-7.3298, 0.63) ccw
  arc A917 (-8.47, 0.63) -> (-8.3213, 0.7604) centre (-8.47, 0.78) ccw
  line L109 (-8.47, 0.63) -> (-8.9893, 0.63)
  arc A918 (-9.138, 0.7604) -> (-8.9893, 0.63) centre (-8.9893, 0.78) ccw
  arc A919 (-9.138, 0.7604) -> (-9.2306, 1.0682) centre (-10.1294, 0.63) ccw
  arc A920 (-9.2306, 1.0682) -> (-9.7296, 1.38) centre (-9.7294, 0.825) ccw
  arc A921 (-9.7296, 1.38) -> (-10.2287, 1.0682) centre (-9.7298, 0.825) ccw
  arc A922 (-10.2287, 1.0682) -> (-10.3213, 0.7604) centre (-9.3298, 0.63) ccw
  arc A923 (-10.47, 0.63) -> (-10.3213, 0.7604) centre (-10.47, 0.78) ccw
  line L110 (-10.47, 0.63) -> (-10.9893, 0.63)
  arc A924 (-11.138, 0.7604) -> (-10.9893, 0.63) centre (-10.9893, 0.78) ccw
  arc A925 (-11.138, 0.7604) -> (-11.2306, 1.0682) centre (-12.1294, 0.63) ccw
  arc A926 (-11.2306, 1.0682) -> (-11.7296, 1.38) centre (-11.7294, 0.825) ccw
  arc A927 (-11.7296, 1.38) -> (-12.2287, 1.0682) centre (-11.7298, 0.825) ccw
  arc A928 (-12.2287, 1.0682) -> (-12.3213, 0.7604) centre (-11.3298, 0.63) ccw
  arc A929 (-12.47, 0.63) -> (-12.3213, 0.7604) centre (-12.47, 0.78) ccw
  line L111 (-12.47, 0.63) -> (-12.9893, 0.63)
  arc A930 (-13.138, 0.7604) -> (-12.9893, 0.63) centre (-12.9893, 0.78) ccw
  arc A931 (-13.138, 0.7604) -> (-13.2306, 1.0682) centre (-14.1294, 0.63) ccw
  arc A932 (-13.2306, 1.0682) -> (-13.7296, 1.38) centre (-13.7294, 0.825) ccw
  arc A933 (-13.7296, 1.38) -> (-14.2287, 1.0682) centre (-13.7298, 0.825) ccw
  arc A934 (-14.2287, 1.0682) -> (-14.3213, 0.7604) centre (-13.3298, 0.63) ccw
  arc A935 (-14.47, 0.63) -> (-14.3213, 0.7604) centre (-14.47, 0.78) ccw
  line L112 (-14.47, 0.63) -> (-14.9893, 0.63)
  arc A936 (-15.138, 0.7604) -> (-14.9893, 0.63) centre (-14.9893, 0.78) ccw
  arc A937 (-15.138, 0.7604) -> (-15.2306, 1.0682) centre (-16.1294, 0.63) ccw
  arc A938 (-15.2306, 1.0682) -> (-15.7296, 1.38) centre (-15.7294, 0.825) ccw
  arc A939 (-15.7296, 1.38) -> (-16.2287, 1.0682) centre (-15.7298, 0.825) ccw
  arc A940 (-16.2287, 1.0682) -> (-16.3213, 0.7604) centre (-15.3298, 0.63) ccw
  arc A941 (-16.47, 0.63) -> (-16.3213, 0.7604) centre (-16.47, 0.78) ccw
  line L113 (-16.47, 0.63) -> (-16.9893, 0.63)
  arc A942 (-17.138, 0.7604) -> (-16.9893, 0.63) centre (-16.9893, 0.78) ccw
  arc A943 (-17.138, 0.7604) -> (-17.2306, 1.0682) centre (-18.1294, 0.63) ccw
  arc A944 (-17.2306, 1.0682) -> (-17.7296, 1.38) centre (-17.7294, 0.825) ccw
  arc A945 (-17.7296, 1.38) -> (-18.2287, 1.0682) centre (-17.7298, 0.825) ccw
  arc A946 (-18.2287, 1.0682) -> (-18.3213, 0.7604) centre (-17.3298, 0.63) ccw
  arc A947 (-18.47, 0.63) -> (-18.3213, 0.7604) centre (-18.47, 0.78) ccw
  line L114 (-18.47, 0.63) -> (-18.9893, 0.63)
  arc A948 (-19.138, 0.7604) -> (-18.9893, 0.63) centre (-18.9893, 0.78) ccw
  arc A949 (-19.138, 0.7604) -> (-19.2306, 1.0682) centre (-20.1294, 0.63) ccw
  arc A950 (-19.2306, 1.0682) -> (-19.7296, 1.38) centre (-19.7294, 0.825) ccw
  arc A951 (-19.7296, 1.38) -> (-20.2287, 1.0682) centre (-19.7298, 0.825) ccw
  arc A952 (-20.2287, 1.0682) -> (-20.3213, 0.7604) centre (-19.3298, 0.63) ccw
  arc A953 (-20.47, 0.63) -> (-20.3213, 0.7604) centre (-20.47, 0.78) ccw
  line L115 (-20.47, 0.63) -> (-20.9893, 0.63)
  arc A954 (-21.138, 0.7604) -> (-20.9893, 0.63) centre (-20.9893, 0.78) ccw
  arc A955 (-21.138, 0.7604) -> (-21.2306, 1.0682) centre (-22.1294, 0.63) ccw
  arc A956 (-21.2306, 1.0682) -> (-21.7296, 1.38) centre (-21.7294, 0.825) ccw
  arc A957 (-21.7296, 1.38) -> (-22.2287, 1.0682) centre (-21.7298, 0.825) ccw
  arc A958 (-22.2287, 1.0682) -> (-22.3213, 0.7604) centre (-21.3298, 0.63) ccw
  arc A959 (-22.47, 0.63) -> (-22.3213, 0.7604) centre (-22.47, 0.78) ccw
  line L116 (-22.47, 0.63) -> (-22.9893, 0.63)
  arc A960 (-23.138, 0.7604) -> (-22.9893, 0.63) centre (-22.9893, 0.78) ccw
  arc A961 (-23.138, 0.7604) -> (-23.2306, 1.0682) centre (-24.1294, 0.63) ccw
  arc A962 (-23.2306, 1.0682) -> (-23.7296, 1.38) centre (-23.7294, 0.825) ccw
  arc A963 (-23.7296, 1.38) -> (-24.2287, 1.0682) centre (-23.7298, 0.825) ccw
  arc A964 (-24.2287, 1.0682) -> (-24.3213, 0.7604) centre (-23.3298, 0.63) ccw
  arc A965 (-24.47, 0.63) -> (-24.3213, 0.7604) centre (-24.47, 0.78) ccw
  line L117 (-24.47, 0.63) -> (-24.9893, 0.63)
  arc A966 (-25.138, 0.7604) -> (-24.9893, 0.63) centre (-24.9893, 0.78) ccw
  arc A967 (-25.138, 0.7604) -> (-25.2306, 1.0682) centre (-26.1294, 0.63) ccw
  arc A968 (-25.2306, 1.0682) -> (-25.7296, 1.38) centre (-25.7294, 0.825) ccw
  arc A969 (-25.7296, 1.38) -> (-26.2287, 1.0682) centre (-25.7298, 0.825) ccw
  arc A970 (-26.2287, 1.0682) -> (-26.3213, 0.7604) centre (-25.3298, 0.63) ccw
  arc A971 (-26.47, 0.63) -> (-26.3213, 0.7604) centre (-26.47, 0.78) ccw
  line L118 (-26.47, 0.63) -> (-26.9893, 0.63)
  arc A972 (-27.138, 0.7604) -> (-26.9893, 0.63) centre (-26.9893, 0.78) ccw
  arc A973 (-27.138, 0.7604) -> (-27.2306, 1.0682) centre (-28.1294, 0.63) ccw
  arc A974 (-27.2306, 1.0682) -> (-27.7296, 1.38) centre (-27.7294, 0.825) ccw
  arc A975 (-27.7296, 1.38) -> (-28.2287, 1.0682) centre (-27.7298, 0.825) ccw
  arc A976 (-28.2287, 1.0682) -> (-28.3213, 0.7604) centre (-27.3298, 0.63) ccw
  arc A977 (-28.47, 0.63) -> (-28.3213, 0.7604) centre (-28.47, 0.78) ccw
  line L119 (-28.47, 0.63) -> (-28.9893, 0.63)
  arc A978 (-29.138, 0.7604) -> (-28.9893, 0.63) centre (-28.9893, 0.78) ccw
  arc A979 (-29.138, 0.7604) -> (-29.2306, 1.0682) centre (-30.1294, 0.63) ccw
  arc A980 (-29.2306, 1.0682) -> (-29.7296, 1.38) centre (-29.7294, 0.825) ccw
  arc A981 (-29.7296, 1.38) -> (-30.2287, 1.0682) centre (-29.7298, 0.825) ccw
  arc A982 (-30.2287, 1.0682) -> (-30.3213, 0.7604) centre (-29.3298, 0.63) ccw
  arc A983 (-30.47, 0.63) -> (-30.3213, 0.7604) centre (-30.47, 0.78) ccw
  line L120 (-30.47, 0.63) -> (-30.9893, 0.63)
  arc A984 (-31.138, 0.7604) -> (-30.9893, 0.63) centre (-30.9893, 0.78) ccw
  arc A985 (-31.138, 0.7604) -> (-31.2306, 1.0682) centre (-32.1294, 0.63) ccw
  arc A986 (-31.2306, 1.0682) -> (-31.7296, 1.38) centre (-31.7294, 0.825) ccw
  arc A987 (-31.7296, 1.38) -> (-32.2287, 1.0682) centre (-31.7298, 0.825) ccw
  arc A988 (-32.2287, 1.0682) -> (-32.3213, 0.7604) centre (-31.3298, 0.63) ccw
  arc A989 (-32.47, 0.63) -> (-32.3213, 0.7604) centre (-32.47, 0.78) ccw
  line L121 (-32.47, 0.63) -> (-32.9893, 0.63)
  arc A990 (-33.138, 0.7604) -> (-32.9893, 0.63) centre (-32.9893, 0.78) ccw
  arc A991 (-33.138, 0.7604) -> (-33.2306, 1.0682) centre (-34.1294, 0.63) ccw
  arc A992 (-33.2306, 1.0682) -> (-33.7296, 1.38) centre (-33.7294, 0.825) ccw
  arc A993 (-33.7296, 1.38) -> (-34.2287, 1.0682) centre (-33.7298, 0.825) ccw
  arc A994 (-34.2287, 1.0682) -> (-34.3213, 0.7604) centre (-33.3298, 0.63) ccw
  arc A995 (-34.47, 0.63) -> (-34.3213, 0.7604) centre (-34.47, 0.78) ccw
  line L122 (-34.47, 0.63) -> (-34.9893, 0.63)
  arc A996 (-35.138, 0.7604) -> (-34.9893, 0.63) centre (-34.9893, 0.78) ccw
  arc A997 (-35.138, 0.7604) -> (-35.2306, 1.0682) centre (-36.1294, 0.63) ccw
  arc A998 (-35.2306, 1.0682) -> (-35.7296, 1.38) centre (-35.7294, 0.825) ccw
  arc A999 (-35.7296, 1.38) -> (-36.2287, 1.0682) centre (-35.7298, 0.825) ccw
  arc A1000 (-36.2287, 1.0682) -> (-36.3213, 0.7604) centre (-35.3298, 0.63) ccw
  arc A1001 (-36.47, 0.63) -> (-36.3213, 0.7604) centre (-36.47, 0.78) ccw
  line L123 (-36.47, 0.63) -> (-36.9893, 0.63)
  arc A1002 (-37.138, 0.7604) -> (-36.9893, 0.63) centre (-36.9893, 0.78) ccw
  arc A1003 (-37.138, 0.7604) -> (-37.2306, 1.0682) centre (-38.1294, 0.63) ccw
  arc A1004 (-37.2306, 1.0682) -> (-37.7296, 1.38) centre (-37.7294, 0.825) ccw
  arc A1005 (-37.7296, 1.38) -> (-38.2287, 1.0682) centre (-37.7298, 0.825) ccw
  arc A1006 (-38.2287, 1.0682) -> (-38.3213, 0.7604) centre (-37.3298, 0.63) ccw
  arc A1007 (-38.47, 0.63) -> (-38.3213, 0.7604) centre (-38.47, 0.78) ccw
  line L124 (-38.47, 0.63) -> (-38.9893, 0.63)
  arc A1008 (-39.138, 0.7604) -> (-38.9893, 0.63) centre (-38.9893, 0.78) ccw
  arc A1009 (-39.138, 0.7604) -> (-39.2306, 1.0682) centre (-40.1294, 0.63) ccw
  arc A1010 (-39.2306, 1.0682) -> (-39.7296, 1.38) centre (-39.7294, 0.825) ccw
  arc A1011 (-39.7296, 1.38) -> (-40.2287, 1.0682) centre (-39.7298, 0.825) ccw
  arc A1012 (-40.2287, 1.0682) -> (-40.3213, 0.7604) centre (-39.3298, 0.63) ccw
  arc A1013 (-40.47, 0.63) -> (-40.3213, 0.7604) centre (-40.47, 0.78) ccw
  line L125 (-40.47, 0.63) -> (-40.9893, 0.63)
  arc A1014 (-41.138, 0.7604) -> (-40.9893, 0.63) centre (-40.9893, 0.78) ccw
  arc A1015 (-41.138, 0.7604) -> (-41.2306, 1.0682) centre (-42.1294, 0.63) ccw
  arc A1016 (-41.2306, 1.0682) -> (-41.7296, 1.38) centre (-41.7294, 0.825) ccw
  arc A1017 (-41.7296, 1.38) -> (-42.2287, 1.0682) centre (-41.7298, 0.825) ccw
  arc A1018 (-42.2287, 1.0682) -> (-42.3213, 0.7604) centre (-41.3298, 0.63) ccw
  arc A1019 (-42.47, 0.63) -> (-42.3213, 0.7604) centre (-42.47, 0.78) ccw
  line L126 (-42.47, 0.63) -> (-42.9893, 0.63)
  arc A1020 (-43.138, 0.7604) -> (-42.9893, 0.63) centre (-42.9893, 0.78) ccw
  arc A1021 (-43.138, 0.7604) -> (-43.2306, 1.0682) centre (-44.1294, 0.63) ccw
  arc A1022 (-43.2306, 1.0682) -> (-43.7296, 1.38) centre (-43.7294, 0.825) ccw
  arc A1023 (-43.7296, 1.38) -> (-44.2287, 1.0682) centre (-43.7298, 0.825) ccw
  arc A1024 (-44.2287, 1.0682) -> (-44.3213, 0.7604) centre (-43.3298, 0.63) ccw
  arc A1025 (-44.47, 0.63) -> (-44.3213, 0.7604) centre (-44.47, 0.78) ccw
  line L127 (-44.47, 0.63) -> (-44.9893, 0.63)
  arc A1026 (-45.138, 0.7604) -> (-44.9893, 0.63) centre (-44.9893, 0.78) ccw
  arc A1027 (-45.138, 0.7604) -> (-45.2306, 1.0682) centre (-46.1294, 0.63) ccw
  arc A1028 (-45.2306, 1.0682) -> (-45.7296, 1.38) centre (-45.7294, 0.825) ccw
  arc A1029 (-45.7296, 1.38) -> (-46.2287, 1.0682) centre (-45.7298, 0.825) ccw
  arc A1030 (-46.2287, 1.0682) -> (-46.3213, 0.7604) centre (-45.3298, 0.63) ccw
  arc A1031 (-46.47, 0.63) -> (-46.3213, 0.7604) centre (-46.47, 0.78) ccw
  line L128 (-46.47, 0.63) -> (-46.9893, 0.63)
  arc A1032 (-47.138, 0.7604) -> (-46.9893, 0.63) centre (-46.9893, 0.78) ccw
  arc A1033 (-47.138, 0.7604) -> (-47.2306, 1.0682) centre (-48.1294, 0.63) ccw
  arc A1034 (-47.2306, 1.0682) -> (-47.7296, 1.38) centre (-47.7294, 0.825) ccw
  arc A1035 (-47.7296, 1.38) -> (-48.2287, 1.0682) centre (-47.7298, 0.825) ccw
  arc A1036 (-48.2287, 1.0682) -> (-48.3213, 0.7604) centre (-47.3298, 0.63) ccw
  arc A1037 (-48.47, 0.63) -> (-48.3213, 0.7604) centre (-48.47, 0.78) ccw
  line L129 (-48.47, 0.63) -> (-48.9893, 0.63)
  arc A1038 (-49.138, 0.7604) -> (-48.9893, 0.63) centre (-48.9893, 0.78) ccw
  arc A1039 (-49.138, 0.7604) -> (-49.2306, 1.0682) centre (-50.1294, 0.63) ccw
  arc A1040 (-49.2306, 1.0682) -> (-49.7296, 1.38) centre (-49.7294, 0.825) ccw
  arc A1041 (-49.7296, 1.38) -> (-50.2287, 1.0682) centre (-49.7298, 0.825) ccw
  arc A1042 (-50.2287, 1.0682) -> (-50.3213, 0.7604) centre (-49.3298, 0.63) ccw
  arc A1043 (-50.47, 0.63) -> (-50.3213, 0.7604) centre (-50.47, 0.78) ccw
  line L130 (-50.47, 0.63) -> (-50.9893, 0.63)
  arc A1044 (-51.138, 0.7604) -> (-50.9893, 0.63) centre (-50.9893, 0.78) ccw
  arc A1045 (-51.138, 0.7604) -> (-51.2306, 1.0682) centre (-52.1294, 0.63) ccw
  arc A1046 (-51.2306, 1.0682) -> (-51.7296, 1.38) centre (-51.7294, 0.825) ccw
  arc A1047 (-51.7296, 1.38) -> (-52.2287, 1.0682) centre (-51.7298, 0.825) ccw
  arc A1048 (-52.2287, 1.0682) -> (-52.3213, 0.7604) centre (-51.3298, 0.63) ccw
  arc A1049 (-52.47, 0.63) -> (-52.3213, 0.7604) centre (-52.47, 0.78) ccw
  line L131 (-52.47, 0.63) -> (-52.9893, 0.63)
  arc A1050 (-53.138, 0.7604) -> (-52.9893, 0.63) centre (-52.9893, 0.78) ccw
  arc A1051 (-53.138, 0.7604) -> (-53.2306, 1.0682) centre (-54.1294, 0.63) ccw
  arc A1052 (-53.2306, 1.0682) -> (-53.7296, 1.38) centre (-53.7294, 0.825) ccw
  arc A1053 (-53.7296, 1.38) -> (-54.2287, 1.0682) centre (-53.7298, 0.825) ccw
  arc A1054 (-54.2287, 1.0682) -> (-54.3213, 0.7604) centre (-53.3298, 0.63) ccw
  arc A1055 (-54.47, 0.63) -> (-54.3213, 0.7604) centre (-54.47, 0.78) ccw
  line L132 (-54.47, 0.63) -> (-54.9893, 0.63)
  arc A1056 (-55.138, 0.7604) -> (-54.9893, 0.63) centre (-54.9893, 0.78) ccw
  arc A1057 (-55.138, 0.7604) -> (-55.2306, 1.0682) centre (-56.1294, 0.63) ccw
  arc A1058 (-55.2306, 1.0682) -> (-55.7296, 1.38) centre (-55.7294, 0.825) ccw
  arc A1059 (-55.7296, 1.38) -> (-56.2287, 1.0682) centre (-55.7298, 0.825) ccw
  arc A1060 (-56.2287, 1.0682) -> (-56.3213, 0.7604) centre (-55.3298, 0.63) ccw
  arc A1061 (-56.47, 0.63) -> (-56.3213, 0.7604) centre (-56.47, 0.78) ccw
  line L133 (-56.47, 0.63) -> (-56.9893, 0.63)
  arc A1062 (-57.138, 0.7604) -> (-56.9893, 0.63) centre (-56.9893, 0.78) ccw
  arc A1063 (-57.138, 0.7604) -> (-57.2306, 1.0682) centre (-58.1294, 0.63) ccw
  arc A1064 (-57.2306, 1.0682) -> (-57.7296, 1.38) centre (-57.7294, 0.825) ccw
  arc A1065 (-57.7296, 1.38) -> (-58.2287, 1.0682) centre (-57.7298, 0.825) ccw
  arc A1066 (-58.2287, 1.0682) -> (-58.3213, 0.7604) centre (-57.3298, 0.63) ccw
  arc A1067 (-58.47, 0.63) -> (-58.3213, 0.7604) centre (-58.47, 0.78) ccw
  line L134 (-58.47, 0.63) -> (-58.9893, 0.63)
  arc A1068 (-59.138, 0.7604) -> (-58.9893, 0.63) centre (-58.9893, 0.78) ccw
  arc A1069 (-59.138, 0.7604) -> (-59.2306, 1.0682) centre (-60.1294, 0.63) ccw
  arc A1070 (-59.2306, 1.0682) -> (-59.7296, 1.38) centre (-59.7294, 0.825) ccw
  arc A1071 (-59.7296, 1.38) -> (-60.2287, 1.0682) centre (-59.7298, 0.825) ccw
  arc A1072 (-60.2287, 1.0682) -> (-60.3213, 0.7604) centre (-59.3298, 0.63) ccw
  arc A1073 (-60.47, 0.63) -> (-60.3213, 0.7604) centre (-60.47, 0.78) ccw
  line L135 (-60.47, 0.63) -> (-60.9893, 0.63)
  arc A1074 (-61.138, 0.7604) -> (-60.9893, 0.63) centre (-60.9893, 0.78) ccw
  arc A1075 (-61.138, 0.7604) -> (-61.2306, 1.0682) centre (-62.1294, 0.63) ccw
  arc A1076 (-61.2306, 1.0682) -> (-61.7296, 1.38) centre (-61.7294, 0.825) ccw
  arc A1077 (-61.7296, 1.38) -> (-62.2287, 1.0682) centre (-61.7298, 0.825) ccw
  arc A1078 (-62.2287, 1.0682) -> (-62.3213, 0.7604) centre (-61.3298, 0.63) ccw
  arc A1079 (-62.47, 0.63) -> (-62.3213, 0.7604) centre (-62.47, 0.78) ccw
  line L136 (-62.47, 0.63) -> (-62.9893, 0.63)
  arc A1080 (-63.138, 0.7604) -> (-62.9893, 0.63) centre (-62.9893, 0.78) ccw
  arc A1081 (-63.138, 0.7604) -> (-63.2306, 1.0682) centre (-64.1294, 0.63) ccw
  arc A1082 (-63.2306, 1.0682) -> (-63.7296, 1.38) centre (-63.7294, 0.825) ccw
  arc A1083 (-63.7296, 1.38) -> (-64.2287, 1.0682) centre (-63.7298, 0.825) ccw
  arc A1084 (-64.2287, 1.0682) -> (-64.3213, 0.7604) centre (-63.3298, 0.63) ccw
  arc A1085 (-64.47, 0.63) -> (-64.3213, 0.7604) centre (-64.47, 0.78) ccw
  line L137 (-64.47, 0.63) -> (-64.9893, 0.63)
  arc A1086 (-65.138, 0.7604) -> (-64.9893, 0.63) centre (-64.9893, 0.78) ccw
  arc A1087 (-65.138, 0.7604) -> (-65.2306, 1.0682) centre (-66.1294, 0.63) ccw
  arc A1088 (-65.2306, 1.0682) -> (-65.7296, 1.38) centre (-65.7294, 0.825) ccw
  arc A1089 (-65.7296, 1.38) -> (-66.2287, 1.0682) centre (-65.7298, 0.825) ccw
  arc A1090 (-66.2287, 1.0682) -> (-66.3213, 0.7604) centre (-65.3298, 0.63) ccw
  arc A1091 (-66.47, 0.63) -> (-66.3213, 0.7604) centre (-66.47, 0.78) ccw
  line L138 (-66.47, 0.63) -> (-66.9893, 0.63)
  arc A1092 (-67.138, 0.7604) -> (-66.9893, 0.63) centre (-66.9893, 0.78) ccw
  arc A1093 (-67.138, 0.7604) -> (-67.2306, 1.0682) centre (-68.1294, 0.63) ccw
  arc A1094 (-67.2306, 1.0682) -> (-67.7296, 1.38) centre (-67.7294, 0.825) ccw
  arc A1095 (-67.7296, 1.38) -> (-68.2287, 1.0682) centre (-67.7298, 0.825) ccw
  arc A1096 (-68.2287, 1.0682) -> (-68.3213, 0.7604) centre (-67.3298, 0.63) ccw
  arc A1097 (-68.47, 0.63) -> (-68.3213, 0.7604) centre (-68.47, 0.78) ccw
  line L139 (-68.47, 0.63) -> (-68.9893, 0.63)
  arc A1098 (-69.138, 0.7604) -> (-68.9893, 0.63) centre (-68.9893, 0.78) ccw
  arc A1099 (-69.138, 0.7604) -> (-69.2306, 1.0682) centre (-70.1294, 0.63) ccw
  arc A1100 (-69.2306, 1.0682) -> (-69.7296, 1.38) centre (-69.7294, 0.825) ccw
  arc A1101 (-69.7296, 1.38) -> (-70.2287, 1.0682) centre (-69.7298, 0.825) ccw
  arc A1102 (-70.2287, 1.0682) -> (-70.3213, 0.7604) centre (-69.3298, 0.63) ccw
  arc A1103 (-70.47, 0.63) -> (-70.3213, 0.7604) centre (-70.47, 0.78) ccw
  line L140 (-70.47, 0.63) -> (-70.9893, 0.63)
  arc A1104 (-71.138, 0.7604) -> (-70.9893, 0.63) centre (-70.9893, 0.78) ccw
  arc A1105 (-71.138, 0.7604) -> (-71.2306, 1.0682) centre (-72.1294, 0.63) ccw
  arc A1106 (-71.2306, 1.0682) -> (-71.7296, 1.38) centre (-71.7294, 0.825) ccw
  arc A1107 (-71.7296, 1.38) -> (-72.2287, 1.0682) centre (-71.7298, 0.825) ccw
  arc A1108 (-72.2287, 1.0682) -> (-72.3213, 0.7604) centre (-71.3298, 0.63) ccw
  arc A1109 (-72.47, 0.63) -> (-72.3213, 0.7604) centre (-72.47, 0.78) ccw
  line L141 (-72.47, 0.63) -> (-72.9893, 0.63)
  arc A1110 (-73.138, 0.7604) -> (-72.9893, 0.63) centre (-72.9893, 0.78) ccw
  arc A1111 (-73.138, 0.7604) -> (-73.2306, 1.0682) centre (-74.1294, 0.63) ccw
  arc A1112 (-73.2306, 1.0682) -> (-73.7296, 1.38) centre (-73.7294, 0.825) ccw
  arc A1113 (-73.7296, 1.38) -> (-74.2287, 1.0682) centre (-73.7298, 0.825) ccw
  arc A1114 (-74.2287, 1.0682) -> (-74.3213, 0.7604) centre (-73.3298, 0.63) ccw
  arc A1115 (-74.47, 0.63) -> (-74.3213, 0.7604) centre (-74.47, 0.78) ccw
  line L142 (-74.47, 0.63) -> (-74.9893, 0.63)
  arc A1116 (-75.138, 0.7604) -> (-74.9893, 0.63) centre (-74.9893, 0.78) ccw
  arc A1117 (-75.138, 0.7604) -> (-75.2306, 1.0682) centre (-76.1294, 0.63) ccw
  arc A1118 (-75.2306, 1.0682) -> (-75.7296, 1.38) centre (-75.7294, 0.825) ccw
  arc A1119 (-75.7296, 1.38) -> (-76.2287, 1.0682) centre (-75.7298, 0.825) ccw
  arc A1120 (-76.2287, 1.0682) -> (-76.3213, 0.7604) centre (-75.3298, 0.63) ccw
  arc A1121 (-76.47, 0.63) -> (-76.3213, 0.7604) centre (-76.47, 0.78) ccw
  line L143 (-76.47, 0.63) -> (-76.9893, 0.63)
  arc A1122 (-77.138, 0.7604) -> (-76.9893, 0.63) centre (-76.9893, 0.78) ccw
  arc A1123 (-77.138, 0.7604) -> (-77.2306, 1.0682) centre (-78.1294, 0.63) ccw
  arc A1124 (-77.2306, 1.0682) -> (-77.7296, 1.38) centre (-77.7294, 0.825) ccw
  arc A1125 (-77.7296, 1.38) -> (-78.2287, 1.0682) centre (-77.7298, 0.825) ccw
  arc A1126 (-78.2287, 1.0682) -> (-78.3213, 0.7604) centre (-77.3298, 0.63) ccw
  arc A1127 (-78.47, 0.63) -> (-78.3213, 0.7604) centre (-78.47, 0.78) ccw
  line L144 (-78.47, 0.63) -> (-78.9893, 0.63)
  arc A1128 (-79.138, 0.7604) -> (-78.9893, 0.63) centre (-78.9893, 0.78) ccw
  arc A1129 (-79.138, 0.7604) -> (-79.2306, 1.0682) centre (-80.1294, 0.63) ccw
  arc A1130 (-79.2306, 1.0682) -> (-79.7296, 1.38) centre (-79.7294, 0.825) ccw
  arc A1131 (-79.7296, 1.38) -> (-80.2287, 1.0682) centre (-79.7298, 0.825) ccw
  arc A1132 (-80.2287, 1.0682) -> (-80.3213, 0.7604) centre (-79.3298, 0.63) ccw
  arc A1133 (-80.47, 0.63) -> (-80.3213, 0.7604) centre (-80.47, 0.78) ccw
  line L145 (-80.47, 0.63) -> (-80.9893, 0.63)
  arc A1134 (-81.138, 0.7604) -> (-80.9893, 0.63) centre (-80.9893, 0.78) ccw
  arc A1135 (-81.138, 0.7604) -> (-81.2306, 1.0682) centre (-82.1294, 0.63) ccw
  arc A1136 (-81.2306, 1.0682) -> (-81.7296, 1.38) centre (-81.7294, 0.825) ccw
  arc A1137 (-81.7296, 1.38) -> (-82.2287, 1.0682) centre (-81.7298, 0.825) ccw
  arc A1138 (-82.2287, 1.0682) -> (-82.3213, 0.7604) centre (-81.3298, 0.63) ccw
  arc A1139 (-82.47, 0.63) -> (-82.3213, 0.7604) centre (-82.47, 0.78) ccw
  line L146 (-82.47, 0.63) -> (-82.9893, 0.63)
  arc A1140 (-83.138, 0.7604) -> (-82.9893, 0.63) centre (-82.9893, 0.78) ccw
  arc A1141 (-83.138, 0.7604) -> (-83.2306, 1.0682) centre (-84.1294, 0.63) ccw
  arc A1142 (-83.2306, 1.0682) -> (-83.7296, 1.38) centre (-83.7294, 0.825) ccw
  arc A1143 (-83.7296, 1.38) -> (-84.2287, 1.0682) centre (-83.7298, 0.825) ccw
  arc A1144 (-84.2287, 1.0682) -> (-84.3213, 0.7604) centre (-83.3298, 0.63) ccw
  arc A1145 (-84.47, 0.63) -> (-84.3213, 0.7604) centre (-84.47, 0.78) ccw
  line L147 (-84.47, 0.63) -> (-84.9893, 0.63)
  arc A1146 (-85.138, 0.7604) -> (-84.9893, 0.63) centre (-84.9893, 0.78) ccw
  arc A1147 (-85.138, 0.7604) -> (-85.2306, 1.0682) centre (-86.1294, 0.63) ccw
  arc A1148 (-85.2306, 1.0682) -> (-85.7296, 1.38) centre (-85.7294, 0.825) ccw
  arc A1149 (-85.7296, 1.38) -> (-86.2287, 1.0682) centre (-85.7298, 0.825) ccw
  arc A1150 (-86.2287, 1.0682) -> (-86.3213, 0.7604) centre (-85.3298, 0.63) ccw
  arc A1151 (-86.47, 0.63) -> (-86.3213, 0.7604) centre (-86.47, 0.78) ccw
  line L148 (-86.47, 0.63) -> (-86.9893, 0.63)
  arc A1152 (-87.138, 0.7604) -> (-86.9893, 0.63) centre (-86.9893, 0.78) ccw
  arc A1153 (-87.138, 0.7604) -> (-87.2306, 1.0682) centre (-88.1294, 0.63) ccw
  arc A1154 (-87.2306, 1.0682) -> (-87.7296, 1.38) centre (-87.7294, 0.825) ccw